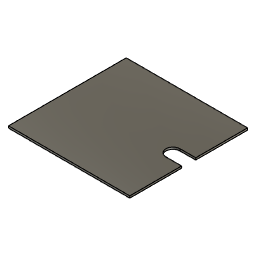
Stack Assembly New with Fixed Holes v4 (Autodesk Fusion 360 archive; units mm, degrees)
design "Floor  1"
Autodesk Fusion 360 part; units mm, degrees
sketch "Sketch1" plane through (0, 0, 0) normal (0, 0, 1) x (1, 0, 0)
  line L0 (-154.5, 150) -> (154.5, 150)
  line L1 (154.5, -150) -> (-154.5, -150)
  line L2 (-154.5, -150) -> (-154.5, 150)
  line L3 (-154.5, 150) -> (154.5, -150) construction
  line L4 (154.5, 18) -> (114.5, 18)
  line L5 (114.5, -18) -> (154.5, -18)
  arc A0 (114.5, 18) -> (114.5, -18) centre (114.5, 0) ccw
  line L6 (154.5, 150) -> (154.5, 18)
  line L7 (154.5, -18) -> (154.5, -150)
  dimension "d1" = 309
  dimension "d2" = 300
  dimension "d6" = 36
  dimension "d7" = 40
  dimension "d8" = 150
  constraint horizontal L0
  constraint vertical L6
  constraint horizontal L1
  constraint vertical L2
  constraint midpoint origin L3
  constraint horizontal L4
  constraint horizontal L5
  constraint collinear L6 L7
  constraint tangent L4 A0
  constraint tangent L5 A0
  measures "d1" distance of L0.start L0.end
  measures "d2" distance of L0.start L1.end
  measures "d6" distance of L4.end L5.start
  measures "d7" distance of L4.start L4.end
  measures "d8" vertical distance of L0.end A0.centre
extrude "Extrude1" add sketch "Sketch1" along normal blind 5

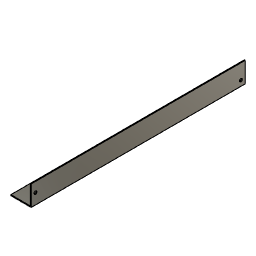
design "Bottom Angle 1.5 inch 400 mm Right"
Autodesk Fusion 360 part; units mm, degrees
sketch "Sketch1" plane through (0, 0, 0) normal (0, 1, 0) x (1, 0, 0)
  line L0 (-38.1, 0) -> (0, 0)
  line L1 (0, 0) -> (0, -38.1)
  line L2 (-38.1, -1.5875) -> (-1.5875, -1.5875)
  line L3 (-1.5875, -1.5875) -> (-1.5875, -38.1)
  line L4 (-1.5875, -38.1) -> (0, -38.1)
  line L5 (-38.1, -1.5875) -> (-38.1, 0)
  dimension "d5" = 38.1
  dimension "d6" = 1.5875
  constraint horizontal L0
  constraint perpendicular L0 L1
  constraint coincident L0.end L1.start
  constraint equal L0 L1
  constraint perpendicular L1 L4
  constraint perpendicular L0 L5
  measures "d5" distance of L0.end L1.end
extrude "Extrude1" add sketch "Sketch1" along normal blind 400
sketch "Sketch3" plane through (-1.5875, 0, 0) normal (-1, 0, 0) x (0, -1, 0)
  line L0 (0, 1.5875) -> (0, 38.1)
  line L1 (0, 38.1) -> (-400, 38.1)
  line L2 (-400, 38.1) -> (-400, 1.5875)
  line L3 (-400, 1.5875) -> (0, 1.5875)
  circle A0 centre (-392, 10) radius 4.9317
  circle A1 centre (-8, 20) radius 5
  line L4 (0, 0) -> (-400, 0)
  dimension "d15" = 10
  dimension "d16" = 8
  dimension "d17" = 8
  dimension "d18" = 20
  measures "d15" distance of A0.centre L4
  measures "d16" distance of L2 A0.centre
  measures "d17" distance of L0 A1.centre
  measures "d18" distance of A1.centre L4
hole "Hole2" at (-1.5875, 8, 20) at (-1.5875, 392, 10) direction (1, 0, 0) diameter 5.5 depth 7 tip angle 118
sketch "Sketch4" plane through (0, 0, 1.5875) normal (0, 0, 1) x (-1, 0, 0)
  line L0 (38.1, 0) -> (1.5875, 0)
  line L1 (1.5875, 0) -> (1.5875, -400)
  line L2 (1.5875, -400) -> (38.1, -400)
  line L3 (38.1, -400) -> (38.1, 0)
  circle A0 centre (19.8375, -34.285) radius 6.9462
  circle A1 centre (19.8375, -365.715) radius 6.9462
  dimension "d22" = 34.285
  dimension "d23" = 34.285
  dimension "d24" = 18.25
  constraint vertical A0.centre A1.centre
  constraint equal A0 A1
  measures "d22" distance of L0 A0.centre
  measures "d23" distance of L2 A1.centre
  measures "d24" distance of L1 A1.centre
hole "Hole3" at (-19.8375, 34.285, 1.5875) at (-19.8375, 365.715, 1.5875) direction (0, 0, -1) diameter 5.5 depth 7 tip angle 118

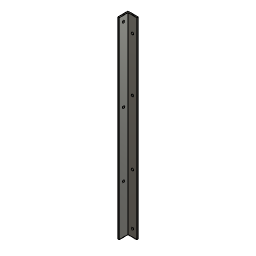
design "angle iron 1 inch 480 mm"
Autodesk Fusion 360 part; units mm, degrees
sketch "Sketch1" plane through (0, 0, 0) normal (0, 1, 0) x (1, 0, 0)
  line L0 (0, 0) -> (25.4, 0)
  line L1 (25.4, 0) -> (25.4, -3.175)
  line L2 (25.4, -3.175) -> (3.175, -3.175)
  line L3 (3.175, -3.175) -> (3.175, -25.4)
  line L4 (3.175, -25.4) -> (0, -25.4)
  line L5 (0, -25.4) -> (0, 0)
  dimension "d1" = 25.4
  dimension "d2" = 25.4
  dimension "d3" = 3.175
  dimension "d4" = 3.175
  constraint coincident L0.start L5.end
  constraint horizontal L0
  constraint perpendicular L0 L1
  constraint perpendicular L1 L2
  constraint perpendicular L0 L3
  constraint perpendicular L3 L4
  constraint perpendicular L0 L5
  measures "d1" distance of L0.start L0.end
  measures "d2" distance of L4.end L0.start
  measures "d3" distance of L3 L5
  measures "d4" distance of L0 L2
extrude "Extrude1" add sketch "Sketch1" along normal blind 480
sketch "Sketch2" plane through (0, 0, 3.175) normal (0, 0, 1) x (1, 0, 0)
  line L0 (3.175, 0) -> (25.4, 0)
  line L1 (25.4, 0) -> (25.4, 480)
  line L2 (25.4, 480) -> (3.175, 480)
  line L3 (3.175, 480) -> (3.175, 0)
  circle A0 centre (14.2875, 18.25) radius 2.75
  circle A1 centre (14.2875, 146.11) radius 2.75
  circle A2 centre (14.2875, 306.51) radius 2.75
  circle A3 centre (14.2875, 440.31) radius 2.75
  line L4 (14.2875, 480) -> (14.2875, 0) construction
  dimension "d7" = 18.25
  dimension "d8" = 146.11
  dimension "d9" = 306.51
  dimension "d10" = 440.31
  dimension "d11" = 5.5
  constraint equal A2 A3
  constraint equal A1 A2
  constraint equal A0 A1
  constraint midpoint L2 L4.start
  constraint midpoint L0 L4.end
  constraint coincident A0.centre L4
  constraint coincident A1.centre L4
  constraint coincident A2.centre L4
  constraint coincident A3.centre L4
  measures "d7" distance of L0 A0.centre
  measures "d8" distance of L0 A1.centre
  measures "d9" distance of L0 A2.centre
  measures "d10" distance of L0 A3.centre
  measures "d11" diameter of A1
sketch "Sketch3" plane through (3.175, 0, 0) normal (1, 0, 0) x (0, 0, -1)
  line L0 (-25.4, 0) -> (-3.175, 0)
  line L1 (-3.175, 0) -> (-3.175, 480)
  line L2 (-3.175, 480) -> (-25.4, 480)
  line L3 (-25.4, 480) -> (-25.4, 0)
  circle A0 centre (-14.2875, 120.71) radius 2.75
  circle A1 centre (-14.2875, 281.11) radius 2.75
  circle A2 centre (-14.2875, 465.71) radius 2.75
  line L4 (-14.2875, 480) -> (-14.2875, 0) construction
  dimension "d12" = 120.71
  dimension "d13" = 5.5
  dimension "d14" = 281.11
  dimension "d15" = 465.71
  constraint equal A1 A2
  constraint equal A0 A1
  constraint midpoint L2 L4.start
  constraint midpoint L0 L4.end
  constraint coincident A2.centre L4
  constraint coincident A1.centre L4
  constraint coincident A0.centre L4
  measures "d12" distance of L0 A0.centre
  measures "d13" diameter of A2
  measures "d14" distance of L0 A1.centre
  measures "d15" distance of L0 A2.centre
hole "Hole1" at (3.175, 465.71, 14.2875) at (3.175, 281.11, 14.2875) at (3.175, 120.71, 14.2875) direction (-1, 0, 0) diameter 5.5 depth 7 tip angle 118
hole "Hole2" at (14.2875, 440.31, 3.175) at (14.2875, 306.51, 3.175) at (14.2875, 146.11, 3.175) at (14.2875, 18.25, 3.175) direction (0, 0, -1) diameter 5.5 depth 7 tip angle 118
equation "d3 = ( 1 / 8 ) * 1 in"
equation "d4 = ( 1 / 8 ) * 1 in"
equation "d8 = 135 mm + 11.11 mm"
equation "d9 = 295.4 mm + 11.11 mm"
equation "d10 = 429.2 mm + 11.11 mm"
equation "d12 = 109.6 mm + 11.11 mm"
equation "d14 = 270 mm + 11.11 mm"
equation "d15 = 454.6 mm + 11.11 mm"

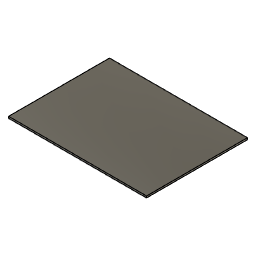
design "Floor  3"
Autodesk Fusion 360 part; units mm, degrees
sketch "Sketch1" plane through (0, 0, 0) normal (0, 0, 1) x (1, 0, 0)
  line L0 (-205, 150) -> (205, 150)
  line L1 (205, 150) -> (205, -150)
  line L2 (205, -150) -> (-205, -150)
  line L3 (-205, -150) -> (-205, 150)
  line L4 (-205, 150) -> (205, -150) construction
  dimension "d1" = 410
  dimension "d2" = 300
  constraint horizontal L0
  constraint vertical L1
  constraint horizontal L2
  constraint vertical L3
  constraint midpoint origin L4
  measures "d1" distance of L0.start L0.end
  measures "d2" distance of L0.start L2.end
extrude "Extrude1" add sketch "Sketch1" along normal blind 5

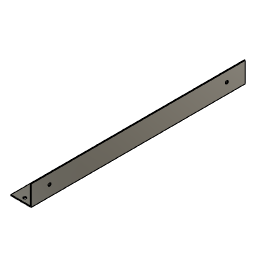
design "Bottom Angle 1.5 inch 400 mm Left"
Autodesk Fusion 360 part; units mm, degrees
sketch "Sketch1" plane through (0, 0, 0) normal (0, 1, 0) x (1, 0, 0)
  line L0 (-38.1, 0) -> (0, 0)
  line L1 (0, 0) -> (0, -38.1)
  line L2 (-38.1, -1.5875) -> (-1.5875, -1.5875)
  line L3 (-1.5875, -1.5875) -> (-1.5875, -38.1)
  line L4 (-1.5875, -38.1) -> (0, -38.1)
  line L5 (-38.1, -1.5875) -> (-38.1, 0)
  dimension "d5" = 38.1
  dimension "d6" = 1.5875
  constraint horizontal L0
  constraint perpendicular L0 L1
  constraint coincident L0.end L1.start
  constraint equal L0 L1
  constraint perpendicular L1 L4
  constraint perpendicular L0 L5
  measures "d5" distance of L0.end L1.end
extrude "Extrude1" add sketch "Sketch1" along normal blind 400
sketch "Sketch2" plane through (0, 0, 1.5875) normal (0, 0, 1) x (-1, 0, 0)
  line L0 (38.1, 0) -> (1.5875, 0)
  line L1 (1.5875, 0) -> (1.5875, -400)
  line L2 (1.5875, -400) -> (38.1, -400)
  line L3 (38.1, -400) -> (38.1, 0)
  circle A0 centre (10, -392) radius 3.6564
  line L4 (0, 0) -> (0, -400)
  circle A1 centre (20, -8) radius 4.5897
  dimension "d7" = 8
  dimension "d9" = 10
  dimension "d10" = 8
  dimension "d11" = 20
  measures "d7" distance of L2 A0.centre
  measures "d9" distance of A0.centre L4
  measures "d10" distance of L0 A1.centre
  measures "d11" distance of L4 A1.centre
hole "Hole1" at (-20, 8, 1.5875) at (-10, 392, 1.5875) direction (0, 0, -1) diameter 5.5 depth 7 tip angle 118
sketch "Sketch3" plane through (-1.5875, 0, 0) normal (-1, 0, 0) x (0, -1, 0)
  line L0 (0, 1.5875) -> (0, 38.1)
  line L1 (0, 38.1) -> (-400, 38.1)
  line L2 (-400, 38.1) -> (-400, 1.5875)
  line L3 (-400, 1.5875) -> (0, 1.5875)
  circle A0 centre (-365.715, 19.8375) radius 7.0711
  circle A1 centre (-34.285, 19.8375) radius 7.0711
  dimension "d15" = 34.285
  dimension "d16" = 34.285
  dimension "d17" = 18.25
  constraint equal A0 A1
  constraint horizontal A0.centre A1.centre
  measures "d15" distance of L2 A0.centre
  measures "d16" distance of L0 A1.centre
  measures "d17" distance of L3 A0.centre
hole "Hole2" at (-1.5875, 34.285, 19.8375) at (-1.5875, 365.715, 19.8375) direction (1, 0, 0) diameter 5.5 depth 7 tip angle 118
equation "d15 = 23.175 mm + 11.11 mm"

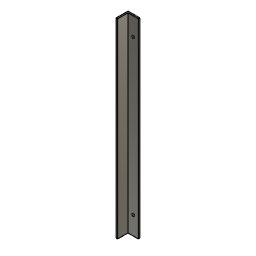
design "angle iron 1 inch 410 mm"
Autodesk Fusion 360 part; units mm, degrees
sketch "Sketch1" plane through (0, 0, 0) normal (0, 0, 1) x (1, 0, 0)
  line L0 (0, 0) -> (25.4, 0)
  line L1 (0, 0) -> (0, -25.4)
  line L2 (3.175, -3.175) -> (25.4, -3.175)
  line L3 (3.175, -3.175) -> (3.175, -25.4)
  line L4 (25.4, 0) -> (25.4, -3.175)
  line L5 (0, -25.4) -> (3.175, -25.4)
  dimension "d1" = 25.4
  dimension "d2" = -3.175
  constraint coincident L0.start L1.start
  constraint horizontal L0
  constraint perpendicular L0 L1
  constraint equal L0 L1
  measures "d1" distance of L0.start L0.end
extrude "Extrude1" add sketch "Sketch1" along normal blind 410
sketch "Sketch2" plane through (0, -3.175, 0) normal (0, -1, 0) x (1, 0, 0)
  line L0 (3.175, 0) -> (25.4, 0)
  line L1 (25.4, 0) -> (25.4, 410)
  line L2 (25.4, 410) -> (3.175, 410)
  line L3 (3.175, 410) -> (3.175, 0)
  circle A0 centre (14.2875, 370.71) radius 4.4166
  circle A1 centre (14.2875, 39.29) radius 4.4166
  line L4 (14.2875, 410) -> (14.2875, 0) construction
  line L5 (14.2875, 205) -> (25.4, 205) construction
  dimension "d6" = 165.71
  dimension "d7" = 165.71
  constraint midpoint L2 L4.start
  constraint midpoint L0 L4.end
  constraint coincident A1.centre L4
  constraint coincident A0.centre L4
  constraint equal A0 A1
  constraint midpoint L4 L5.start
  constraint midpoint L1 L5.end
  measures "d6" distance of A1.centre L5.start
  measures "d7" distance of A0.centre L5.start
hole "Hole1" at (14.2875, -3.175, 370.71) at (14.2875, -3.175, 39.29) direction (0, 1, 0) diameter 5.5 depth 7 tip angle 118

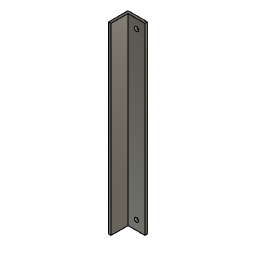
design "angle iron 1 inch 240 mm"
Autodesk Fusion 360 part; units mm, degrees
sketch "Sketch1" plane through (0, 0, 0) normal (0, 0, 1) x (1, 0, 0)
  line L0 (0, 0) -> (25.4, 0)
  line L1 (0, 0) -> (0, -25.4)
  line L2 (3.175, -3.175) -> (25.4, -3.175)
  line L3 (3.175, -3.175) -> (3.175, -25.4)
  line L4 (25.4, 0) -> (25.4, -3.175)
  line L5 (0, -25.4) -> (3.175, -25.4)
  dimension "d1" = 25.4
  dimension "d2" = -3.175
  constraint coincident L0.start L1.start
  constraint horizontal L0
  constraint perpendicular L0 L1
  constraint equal L0 L1
  measures "d1" distance of L0.start L0.end
extrude "Extrude1" add sketch "Sketch1" along normal blind 240
sketch "Sketch2" plane through (0, -3.175, 0) normal (0, -1, 0) x (1, 0, 0)
  line L0 (3.175, 0) -> (25.4, 0)
  line L1 (25.4, 0) -> (25.4, 240)
  line L2 (25.4, 240) -> (3.175, 240)
  line L3 (3.175, 240) -> (3.175, 0)
  circle A0 centre (14.2875, 228) radius 2.75
  circle A1 centre (14.2875, 12) radius 2.75
  line L4 (14.2875, 240) -> (14.2875, 0) construction
  dimension "d5" = 5.5
  dimension "d6" = 12
  dimension "d7" = 12
  constraint equal A0 A1
  constraint midpoint L2 L4.start
  constraint midpoint L0 L4.end
  constraint coincident A1.centre L4
  constraint coincident A0.centre L4
  measures "d5" diameter of A0
  measures "d6" distance of L2 A0.centre
  measures "d7" distance of L0 A1.centre
hole "Hole1" at (14.2875, -3.175, 12) at (14.2875, -3.175, 228) direction (0, 1, 0) diameter 5.5 depth 7 tip angle 118

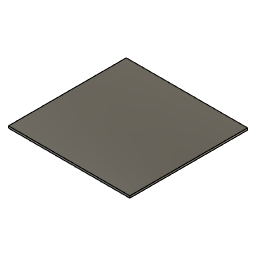
design "Floor  2"
Autodesk Fusion 360 part; units mm, degrees
sketch "Sketch1" plane through (0, 0, 0) normal (0, 0, 1) x (1, 0, 0)
  line L0 (-154.5, 150) -> (154.5, 150)
  line L1 (154.5, 150) -> (154.5, -150)
  line L2 (154.5, -150) -> (-154.5, -150)
  line L3 (-154.5, -150) -> (-154.5, 150)
  line L4 (-154.5, 150) -> (154.5, -150) construction
  dimension "d1" = 309
  dimension "d2" = 300
  constraint horizontal L0
  constraint vertical L1
  constraint horizontal L2
  constraint vertical L3
  constraint midpoint origin L4
  measures "d1" distance of L0.start L0.end
  measures "d2" distance of L0.start L2.end
extrude "Extrude1" add sketch "Sketch1" along normal blind 5

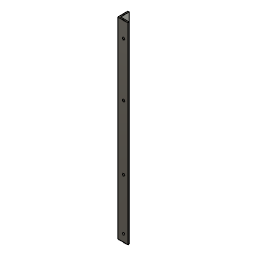
design "angle iron 1 inch 480 mm Opposite"
Autodesk Fusion 360 part; units mm, degrees
sketch "Sketch1" plane through (0, 0, 0) normal (0, 1, 0) x (1, 0, 0)
  line L0 (0, 0) -> (25.4, 0)
  line L1 (25.4, 0) -> (25.4, -3.175)
  line L2 (25.4, -3.175) -> (3.175, -3.175)
  line L3 (3.175, -3.175) -> (3.175, -25.4)
  line L4 (3.175, -25.4) -> (0, -25.4)
  line L5 (0, -25.4) -> (0, 0)
  dimension "d1" = 25.4
  dimension "d2" = 25.4
  dimension "d3" = 3.175
  dimension "d4" = 3.175
  constraint coincident L0.start L5.end
  constraint horizontal L0
  constraint perpendicular L0 L1
  constraint perpendicular L1 L2
  constraint perpendicular L0 L3
  constraint perpendicular L3 L4
  constraint perpendicular L0 L5
  measures "d1" distance of L0.start L0.end
  measures "d2" distance of L4.end L0.start
  measures "d3" distance of L3 L5
  measures "d4" distance of L0 L2
extrude "Extrude1" add sketch "Sketch1" along normal blind 480 makes body 1
sketch "Sketch2" plane through (0, 0, 3.175) normal (0, 0, 1) x (1, 0, 0)
  line L0 (3.175, 0) -> (25.4, 0)
  line L1 (25.4, 0) -> (25.4, 480)
  line L2 (25.4, 480) -> (3.175, 480)
  line L3 (3.175, 480) -> (3.175, 0)
  circle A0 centre (14.2875, 18.25) radius 2.75
  circle A1 centre (14.2875, 146.11) radius 2.75
  circle A2 centre (14.2875, 306.51) radius 2.75
  circle A3 centre (14.2875, 440.31) radius 2.75
  line L4 (14.2875, 480) -> (14.2875, 0) construction
  dimension "d7" = 18.25
  dimension "d8" = 146.11
  dimension "d9" = 306.51
  dimension "d10" = 440.31
  dimension "d11" = 5.5
  constraint equal A2 A3
  constraint equal A1 A2
  constraint equal A0 A1
  constraint midpoint L2 L4.start
  constraint midpoint L0 L4.end
  constraint coincident A0.centre L4
  constraint coincident A1.centre L4
  constraint coincident A2.centre L4
  constraint coincident A3.centre L4
  measures "d7" distance of L0 A0.centre
  measures "d8" distance of L0 A1.centre
  measures "d9" distance of L0 A2.centre
  measures "d10" distance of L0 A3.centre
  measures "d11" diameter of A1
sketch "Sketch3" plane through (3.175, 0, 0) normal (1, 0, 0) x (0, 0, -1)
  line L0 (-25.4, 0) -> (-3.175, 0)
  line L1 (-3.175, 0) -> (-3.175, 480)
  line L2 (-3.175, 480) -> (-25.4, 480)
  line L3 (-25.4, 480) -> (-25.4, 0)
  circle A0 centre (-14.2875, 120.71) radius 2.75
  circle A1 centre (-14.2875, 281.11) radius 2.75
  circle A2 centre (-14.2875, 465.71) radius 2.75
  line L4 (-14.2875, 480) -> (-14.2875, 0) construction
  dimension "d12" = 120.71
  dimension "d13" = 5.5
  dimension "d14" = 281.11
  dimension "d15" = 465.71
  constraint equal A1 A2
  constraint equal A0 A1
  constraint midpoint L2 L4.start
  constraint midpoint L0 L4.end
  constraint coincident A2.centre L4
  constraint coincident A1.centre L4
  constraint coincident A0.centre L4
  measures "d12" distance of L0 A0.centre
  measures "d13" diameter of A2
  measures "d14" distance of L0 A1.centre
  measures "d15" distance of L0 A2.centre
hole "Hole1" at (3.175, 465.71, 14.2875) at (3.175, 281.11, 14.2875) at (3.175, 120.71, 14.2875) direction (-1, 0, 0) diameter 5.5 depth 7 tip angle 118 bodies 1
hole "Hole2" at (14.2875, 440.31, 3.175) at (14.2875, 306.51, 3.175) at (14.2875, 146.11, 3.175) at (14.2875, 18.25, 3.175) direction (0, 0, -1) diameter 5.5 depth 7 tip angle 118 bodies 1
mirror "Mirror1" about plane through (0, 0, 0) normal (0, 0, 1) of bodies 1 merged
split "Split1" by plane through (0, 0, 0) normal (0, 0, 1) bodies 1 makes body 2 at (0, 39.3339, 13.07)
hidden bodies 2
equation "d3 = ( 1 / 8 ) * 1 in"
equation "d4 = ( 1 / 8 ) * 1 in"
equation "d8 = 135 mm + 11.11 mm"
equation "d9 = 295.4 mm + 11.11 mm"
equation "d10 = 429.2 mm + 11.11 mm"
equation "d12 = 109.6 mm + 11.11 mm"
equation "d14 = 270 mm + 11.11 mm"
equation "d15 = 454.6 mm + 11.11 mm"
